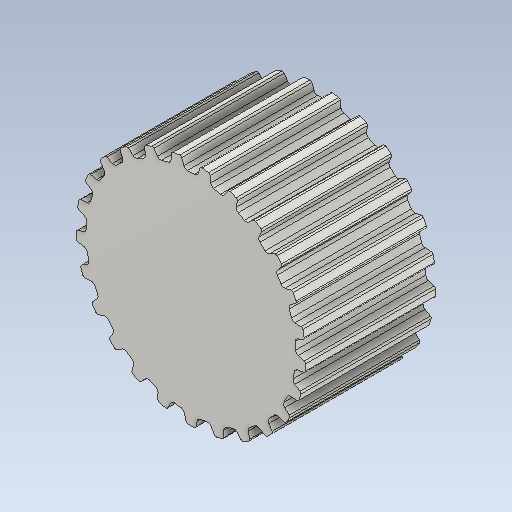
# Autodesk Inventor part: Synchronous Pulley1
Saved by Autodesk Inventor 2020.3 (Build 243373000, 373)
## iProperties
CustomPartVersion: 1
Created: 2022-07-01
Part Number: Synchronous Pulley1
Material: Steel
Document SubType Name: Modeling
Designer: karimi2
Density: 7.85 g/cm^3
Appearance: Steel
Mass: 12.1789 g
Surface Area: 9.57907 cm^2
Volume: 1.55146 cm^3
Author: karimi2
Autodesk Inventor part; units mm, degrees
ref_plane "YZ Plane" through (0, 0, 0) normal (1, 0, 0) x (0, 1, 0)
ref_plane "XZ Plane" through (0, 0, 0) normal (0, 1, 0) x (-1, 0, 0)
ref_plane "XY Plane" through (0, 0, 0) normal (0, 0, 1) x (1, 0, 0)
sketch "Pulley Sketch" plane through (0, 0, 0) normal (0, 0, 1) x (1, 0, 0)
  circle A0 centre (0, 0) radius 8.0851 construction
  circle A1 centre (0, 0) radius 7.8311
  circle A2 centre (0, 0) radius 7.1453
  line L0 (-0.6586, 7.8033) -> (-0.4191, 7.1453)
  line L1 (-0.4191, 7.1453) -> (0.4191, 7.1453)
  line L2 (0.4191, 7.1453) -> (0.6586, 7.8033)
  line L3 (0, 0) -> (0, 7.8311) construction
  point P0 (0, 7.1453)
  dimension "d0" = 16.1701
  dimension "d1" = 0.254
  dimension "d2" = 0.6858
  dimension "d3" = 40
  dimension "d4" = 0.8382
  constraints: 8 end point, 3 coincident, 3 point on circle, 2 centre point, 1 horizontal, 1 midpoint, 1 point on line, 1 vertical, 1 vertical alignment, 3 other
  measures "d0" diameter of A0
  measures "d1" radial gap between concentric circles of A0 A1
  measures "d3" angle of L2 L0
  measures "d4" distance of L0.end L1.end
extrude "Base Body" add sketch "Pulley Sketch" along normal mid plane 8.89 contours A2 | A1 L0 L1 L2 | L2 L1 L0 A1
extrude "Tooth" cut sketch "Pulley Sketch" along normal through all both and the other way through all contours L2 L1 L0 A1 picked at (0, 7.6004)
fillet "Tooth Fillet" radius 0.254 2 edges at (0.4191, 7.1453, 0) (-0.4191, 7.1453, 0)
fillet "Tooth Fillet" radius 0.127 4 edges at (-0.6586, 7.8033, 2.2225) (-0.6586, 7.8033, -2.2225) (0.6586, 7.8033, 2.2225) (0.6586, 7.8033, -2.2225)
pattern_circular "Teeth" count 25 over 360 about axis through (0, 0, -10) along (0, 0, 1) of "Tooth", "Tooth Fillet"
feature "Left flange" [suppressed]
feature "Right flange" [suppressed]
equation "\"d1\" = da_a"
equation "\"d2\" = da_hg"
equation "\"d3\" = 2 * da_fi"
equation "\"d4\" = da_bw"
equation "\"d5\" = da_bf"
equation "\"d7\" = da_bf"
equation "\"d9\" = da_rb"
equation "\"d10\" = da_rt"
equation "\"da_pb\" = 2.032"
equation "\"da_fi\" = 20deg"
equation "\"da_hg\" = 0.6858"
equation "\"da_bw\" = 0.8382"
equation "\"da_rb\" = 0.254"
equation "\"da_rt\" = 0.127"
equation "\"da_a\" = 0.254"
equation "\"da_bf\" = 8.89"
equation "\"da_wf\" = 1.5"
equation "\"da_hf\" = 1.5"
body "Solid1"
